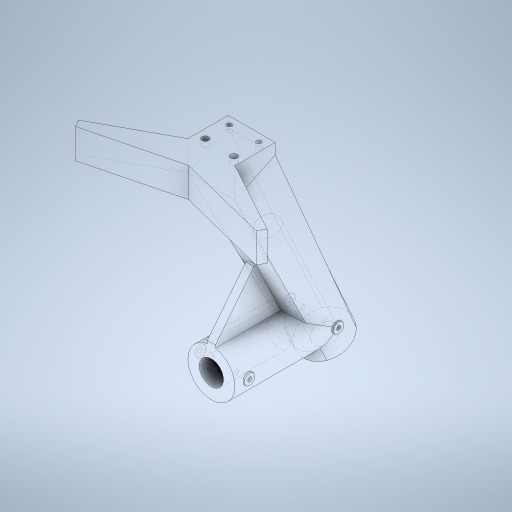
# Autodesk Inventor part: UpperLandingLegMount
Saved by Autodesk Inventor 2023 (Build 270158000, 158)
## iProperties
Created: 2022-12-13
Part Number: UpperLandingLegMount
Material: Generic
Document SubType Name: Modeling
Designer: ethan
Density: 1 g/cm^3
Appearance: Default
Author: ethan
Autodesk Inventor part; units mm, degrees
ref_plane "YZ Plane" through (0, 0, 0) normal (1, 0, 0) x (0, 1, 0)
ref_plane "XZ Plane" through (0, 0, 0) normal (0, 1, 0) x (-1, 0, 0)
sketch "Sketch1" plane through (0, 0, 0) normal (0, 1, 0) x (-1, 0, 0)
  circle A0 centre (5.75, 0) radius 1.35 construction
  circle A1 centre (5.75, 0) radius 1.75
  circle A2 centre (24.25, 0) radius 1.55 construction
  circle A3 centre (24.25, 0) radius 2.5
  circle A4 centre (23.5, 22) radius 1.55 construction
  circle A5 centre (23.5, 22) radius 2.5
  circle A6 centre (5.75, 22) radius 1.35 construction
  circle A7 centre (5.75, 22) radius 1.75
  line L0 (5.75, 0) -> (0, 0) construction
  line L1 (0, 35.2322) -> (0, -14.7678) construction
  line L2 (5.75, 22) -> (24.25, 22) construction
  line L3 (24.25, 22) -> (24.25, 0) construction
  line L4 (24.25, 0) -> (5.75, 0) construction
  line L5 (5.75, 0) -> (5.75, 22) construction
  line L6 (0, -6.5) -> (30, -6.5)
  line L7 (30, -6.5) -> (30, 28.5)
  line L8 (30, 28.5) -> (0, 28.5)
  line L9 (0, 28.5) -> (0, -6.5)
  line L10 (30, 28.5) -> (30, 28.5)
  line L11 (30, 28.5) -> (58.7655, 81.155)
  line L12 (58.7655, 81.155) -> (64.031, 78.2784)
  line L13 (64.031, 78.2784) -> (30, 15.985)
  line L14 (30, 11) -> (0, 11) construction
  line L15 (30, -6.5) -> (58.7655, -59.155)
  line L16 (58.7655, -59.155) -> (64.031, -56.2784)
  line L17 (64.031, -56.2784) -> (30, 6.015)
  point P0 (0, 0)
  point P1 (15, -92.5)
  point P2 (30, 6.015)
  point P3 (30, -6.5)
  dimension "d0" = 3.5
  dimension "d1" = 5
  dimension "d2" = 5
  dimension "d3" = 3.5
  dimension "d4" = 30
  dimension "d5" = 35
  dimension "d6" = 6.5
  dimension "d7" = 22
  dimension "d8" = 18.5
  dimension "d9" = 0
  dimension "d10" = 0
  dimension "d12" = 5.75
  dimension "d13" = 0
  dimension "d14" = 0
  dimension "d64" = 0
  dimension "d65" = 60
  dimension "d66" = 61.352
  dimension "d67" = 6
  dimension "d68" = 90
  dimension "d69" = 90
  constraints: 36 end point, 8 centre point, 4 coincident, 4 parallel, 4 point on line, 4 symmetric about line, 3 horizontal, 3 perpendicular, 2 midpoint
  measures "d0" diameter of A1
  measures "d1" diameter of A3
  measures "d2" diameter of A5
  measures "d3" diameter of A7
  measures "d4" distance of L6.start L6.end
  measures "d5" distance of L6.end L7.end
  measures "d6" distance from line of L6 A3.centre
  measures "d7" distance of L2.end L3.end
  measures "d8" distance of L3.end L4.end
  measures "d9" vertical distance of A3.centre A1.centre
  measures "d10" vertical distance of point (0, 0) A1.centre
  measures "d12" distance from line of L1 A1.centre
  measures "d13" horizontal distance of L2.start A1.centre
  measures "d14" distance from line of L1 point (0, 0)
  measures "d64" distance of L7.end L10.end
  measures "d65" distance of L10.end L11.end
  measures "d66" angle of L10 L11
  measures "d67" distance of L11.end L12.end
  measures "d68" angle of L11 L12
  measures "d69" angle of L12 L13
extrude "Extrusion1" add sketch "Sketch1" along normal blind 4
sketch "Sketch2" plane through (0, 4, 0) normal (0, 1, 0) x (1, 0, 0)
  line L0 (-30, -6.015) -> (-30, -15.985) projected
  line L1 (-30, 6.5) -> (0, 6.5)
  line L2 (0, 6.5) -> (0, -28.5)
  line L3 (0, -28.5) -> (-30, -28.5)
  line L4 (-30, -28.5) -> (-30, 6.5)
  point P0 (0, 0)
  constraints: 8 end point, 2 parallel, 1 horizontal, 1 perpendicular
extrude "Extrusion2" add sketch "Sketch2" along normal blind 4
draft "FaceDraft1" angle 25 pull direction (1, 0, 0) faces at (-10, 8, 16.8333) fixed edges at (0, 8, 11)
ref_plane "Work Plane1" through (67.6189, 153.0092, 28.5) normal (0.4226183, 0.9063078, 0) x (0.9063078, -0.4226183, 0)
sketch "Sketch5" plane through (67.6189, 153.0092, 28.5) normal (0.4226183, 0.9063078, 0) x (0.9063078, -0.4226183, 0)
  line L0 (3.3809, 35) -> (0, 35) construction
  line L1 (-23.8083, 0) -> (-33.1013, 0) construction
  line L2 (3.3809, 35) -> (-33.1013, 0) construction
  circle A0 centre (-14.8602, 17.5) radius 17.5
  point P0 (3.3809, 28.5)
  dimension "d29" = 35
  constraints: 2 end point, 1 centre point, 1 midpoint
  measures "d29" diameter of A0
loft "Loft1" add profiles "Sketch5" section 1 edges at (0, 8, 11) (-15, 14.9946, -6.5) (-30, 21.9892, 11) (-15, 14.9946, 28.5)
sketch "Sketch7" plane through (-30, 0, -6.5) normal (-1, 0, 0) x (0, 0, 1)
  arc A0 (17.5, 124.4892) -> (20.5, 124.7483) centre (17.5, 141.9892) ccw construction
  line L0 (0, 21.9892) -> (35, 21.9892) projected
  line L1 (17.5, 124.4892) -> (17.5, 126.4892) construction
  line L2 (17.5, 126.4892) -> (20.5, 126.4892) construction
  line L3 (20.5, 126.4892) -> (17.5, 126.4892) construction
  line L4 (14.5, 126.4892) -> (14.5, 124.7483) construction
  line L5 (14.5, 86.4892) -> (20.5, 86.4892)
  line L6 (20.5, 86.4892) -> (20.5, 124.7483)
  arc A1 (14.5, 124.7483) -> (17.5, 124.4892) centre (17.5, 141.9892) ccw construction
  arc A2 (20.5, 124.7483) -> (14.5, 124.7483) centre (17.5, 141.9892) ccw
  line L7 (20.5, 124.7483) -> (20.5, 126.4892) construction
  line L8 (17.5, 126.4892) -> (14.5, 126.4892) construction
  line L9 (14.5, 124.7483) -> (14.5, 86.4892)
  point P0 (6.5, 0)
  dimension "d37" = 35
  dimension "d38" = 120
  dimension "d39" = 17.5
  dimension "d40" = 35
  dimension "d57" = 2
  dimension "d58" = 3
  dimension "d59" = 6
  dimension "d60" = 40
  constraints: 18 end point, 6 parallel, 6 point on circle, 5 perpendicular, 3 centre point, 2 horizontal, 1 vertical
  measures "d37" diameter of A0
  measures "d38" distance from line of L0 A0.centre
  measures "d39" horizontal distance of L0.start A0.centre
  measures "d40" distance of L0.start L0.end
  measures "d57" distance of L1.start L1.end
  measures "d58" distance of L1.end L2.end
  measures "d59" distance of L5.end L5.start
  measures "d60" distance of L5.start L4.start
extrude "Extrusion6" add sketch "Sketch7" against normal up to next
sketch "Sketch6" plane through (54.151, 159.2894, 11) normal (0.4226183, 0.9063078, 0) x (0.9063078, -0.4226183, 0)
  circle A0 centre (0, 0) radius 8
  point P0 (18.2411, 11)
  dimension "d34" = 16
  constraints: 1 centre point
  measures "d34" diameter of A0
extrude "Extrusion5" cut sketch "Sketch6" against normal blind 100
sketch "Sketch8" plane through (-30, 141.9892, 11) normal (-1, 0, 0) x (0, 0, 1)
  circle A0 centre (0, 0) radius 9
  point P0 (-11, -141.9892)
  dimension "d43" = 18
  constraints: 1 centre point
  measures "d43" diameter of A0
extrude "Extrusion7" cut sketch "Sketch8" against normal blind 50
sketch "Sketch9" plane through (0, 0, -6.5) normal (0, 0, -1) x (-1, 0, 0)
  line L0 (30, 150.9892) -> (30, 132.9892) projected
  line L1 (30, 141.9892) -> (20, 141.9892) construction
  circle A0 centre (20, 141.9892) radius 4
  line L2 (20, 141.9892) -> (-54.9108, 141.9892) construction
  line L3 (-61.4015, 155.9085) -> (-19.1396, 65.2777) construction
  line L4 (-54.9108, 141.9892) -> (-40.4099, 148.7511) construction
  line L5 (-46.9005, 162.6704) -> (-4.6387, 72.0396) construction
  line L6 (-47.6604, 145.3702) -> (-46.0838, 141.9892) construction
  circle A1 centre (-46.0838, 141.9892) radius 4
  point P0 (0, 0)
  dimension "d46" = 10
  dimension "d47" = 8
  dimension "d50" = 8
  constraints: 8 end point, 3 point on line, 2 centre point, 2 coincident, 2 horizontal, 2 midpoint, 1 perpendicular
  measures "d46" distance of L1.start L1.end
  measures "d47" diameter of A0
  measures "d50" diameter of A1
extrude "Extrusion8" add sketch "Sketch9" along normal mid plane 2
sketch "Sketch10" plane through (-30, 0, 28.5) normal (0, 0, 1) x (1, 0, 0)
  circle A0 centre (10, 141.9892) radius 4 projected
  circle A1 centre (10, 141.9892) radius 4
  circle A2 centre (76.0838, 141.9892) radius 4 projected
  circle A3 centre (76.0838, 141.9892) radius 4
  point P0 (30, 0)
  constraints: 2 centre point, 2 coincident
extrude "Extrusion9" add sketch "Sketch10" along normal mid plane 2
sketch "Sketch11" plane through (-20, 141.9892, -7.5) normal (0, 0, -1) x (-1, 0, 0)
  circle A0 centre (0, 0) radius 1.5
  circle A1 centre (-66.0838, 0) radius 4 projected
  circle A2 centre (-66.0838, 0) radius 1.5
  point P0 (-20, -141.9892)
  dimension "d53" = 3
  dimension "d54" = 3
  constraints: 2 centre point, 1 coincident
  measures "d53" diameter of A0
  measures "d54" diameter of A2
extrude "Extrusion10" cut sketch "Sketch11" against normal through all contours A0 | A2
chamfer "Chamfer1" distance 36.25 distance2 28.575 1 edges at (-30, 86.4892, 11) measured on face at (-30, 86.9892, 11)
sketch "Sketch12" plane through (0, 4, 0) normal (0, 1, 0) x (1, 0, 0)
  point P0 (0, 0)
sketch "Sketch13" plane through (0, 4, 0) normal (0, 1, 0) x (1, 0, 0)
  point P0 (0, 0)
sketch "Sketch15" plane through (0, 0, 0) normal (0, -1, 0) x (1, 0, 0)
  line L0 (-30, -6.5) -> (-58.7655, -59.155) projected
  line L1 (-58.7655, -59.155) -> (-30, -6.5)
  line L2 (-30, -6.5) -> (-30, 28.5)
  line L3 (-30, 28.5) -> (42.0838, 28.5) projected
  line L4 (-64.031, 78.2784) -> (-58.7655, 81.155) projected
  line L5 (-58.7655, 81.155) -> (-30, 28.5) projected
  line L6 (-58.7655, 81.155) -> (-30, 28.5)
  line L7 (-30, 15.985) -> (-64.031, 78.2784) projected
  line L8 (-58.7655, 81.155) -> (-64.031, 78.2784)
  line L9 (-64.031, -56.2784) -> (-58.7655, -59.155)
  line L10 (-30, -6.5) -> (-30, 28.5) construction
  line L11 (-30, 11) -> (-64.031, 11) construction
  line L12 (-47.0155, 11) -> (-64.031, 78.2784)
  line L13 (-64.031, -56.2784) -> (-30, 6.015) projected
  line L14 (-47.0155, 11) -> (-64.031, -56.2784)
  point P0 (0, 0)
  constraints: 16 end point, 2 collinear, 2 midpoint, 1 perpendicular, 1 point on line, 1 vertical
extrude "Extrusion11" add sketch "Sketch15" against normal blind 22
equation "\"d6\" = -0.5 * d7 + 0.5 * d5"
equation "\"d12\" = -0.5 * d8 + 0.5 * d4"
equation "\"d39\" = 0.5 * d40"
body "Solid1"
